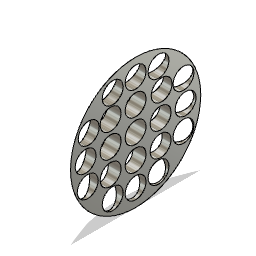
OsmoPod - ZipTie (Autodesk Fusion 360 archive; units mm, degrees)
design "Screen_Cover_12mm"
Autodesk Fusion 360 part; units mm, degrees
sketch "Sketch1" plane through (0, 0, 0) normal (0, 1, 0) x (1, 0, 0)
  line L0 (0, 0) -> (0, 15.875)
  line L1 (0, 0) -> (0, 7.9375)
  line L2 (6.0148, 7.9375) -> (-8.89, 7.9375)
  line L3 (0, 7.9375) -> (-0.254, 7.9375)
  line L4 (0, 7.9375) -> (-1.905, 7.9375)
  line L5 (-1.905, 7.9903) -> (-1.905, 3.048)
  arc A0 (0, 15.875) -> (0, 0) centre (15.584, 7.9375) ccw
  dimension "d1" = 15.875
  dimension "d2" = 1.905
  constraint coincident L0.start L1.start
  constraint vertical L0
  constraint midpoint L0 L1.end
  constraint perpendicular L0 L2
  constraint coincident L2 L3.end
  constraint perpendicular L0 L3
  constraint coincident L2 L4.end
  constraint perpendicular L4 L5
  constraint coincident L4.end A0
  constraint tangent L5 A0
  measures "d1" distance of L0.start L0.end
  measures "d2" distance of L1.end L4.end
revolve "Revolve1" add sketch "Sketch1" angle 360 about axis through (6.0148, 0, -7.9375) along (-1, 0, 0) contours L0 L2 L3 L4 L5 A0
ref_plane "WorkPlane1" through (-2.54, 0, -7.9375) normal (1, 0, 0) x (0, 0, -1)
sketch "Sketch3" plane through (0, 0, 0) normal (1, 0, 0) x (0, 0, -1)
  circle A0 centre (7.9375, 0) radius 7.9375
  circle A1 centre (7.9375, 0) radius 1.2749
  circle A2 centre (7.9375, 2.921) radius 1.2749
  circle A3 centre (7.9375, 5.842) radius 1.2749
  circle A4 centre (7.9375, -2.921) radius 1.2749
  circle A5 centre (7.9375, -5.842) radius 1.2749
  circle A6 centre (10.9855, 0) radius 1.2749
  circle A7 centre (4.8895, 0) radius 1.2749
  circle A8 centre (1.8415, 0) radius 1.2749
  circle A9 centre (14.0335, 0) radius 1.2749
  circle A10 centre (4.8895, 2.921) radius 1.2749
  circle A11 centre (11.1125, 2.921) radius 1.2749
  circle A12 centre (4.8895, -2.921) radius 1.2749
  circle A13 centre (10.9855, -2.921) radius 1.2749
  circle A14 centre (2.2225, 2.794) radius 1.2749
  circle A15 centre (5.1435, 5.588) radius 1.2749
  circle A16 centre (10.7315, 5.588) radius 1.2749
  circle A17 centre (13.7795, 2.794) radius 1.2749
  circle A18 centre (5.1435, -5.588) radius 1.2749
  circle A19 centre (2.0955, -2.794) radius 1.2749
  circle A20 centre (13.7795, -2.794) radius 1.2749
  circle A21 centre (10.7315, -5.588) radius 1.2749
  constraint concentric A0 A1
extrude "Extrude2" cut sketch "Sketch3" against normal blind 3.81 contours A1 | A2 | A3 | A4 | A5 | A6 | A7 | A8 | A9 | A10 | A11 | A12 | A13 | A14 | A15 | A16 | A17 | A18 | A19 | A20 | A21

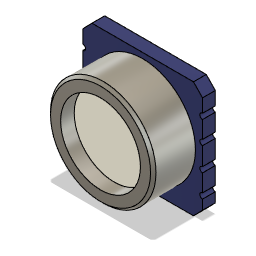
design "MS5803-02BA Package"
Autodesk Fusion 360 part; units mm, degrees
sketch "Sketch1" plane through (0, 0, 0) normal (0, 0, 1) x (1, 0, 0)
  line L0 (2.8, 3.2) -> (-2.8, 3.2)
  line L1 (-2.8, -3.2) -> (2.8, -3.2)
  line L2 (3.0423, 2.9501) -> (-3.0423, -2.9501) construction
  line L3 (-3.0423, 2.9501) -> (3.0423, -2.9501) construction
  circle A0 centre (0, 0) radius 2.2
  line L4 (-2.8, 3.2) -> (-3.3, 2.6844)
  line L5 (3.3, 0) -> (-3.3, 0) construction
  line L6 (0, 3.2) -> (0, -3.2) construction
  line L7 (2.8, 3.2) -> (3.3, 2.6844)
  line L8 (-2.8, -3.2) -> (-3.3, -2.6844)
  line L9 (2.8, -3.2) -> (3.3, -2.6844)
  circle A1 centre (0, 0) radius 2.9075
  line L10 (-2.8, -3.2) -> (-3.3, -3.2) construction
  line L11 (-3.3, -3.2) -> (-3.3, -2) construction
  line L12 (-3.3, -2) -> (-3.3, -0.75) construction
  line L13 (-3.3, -0.75) -> (-3.3, 0.55) construction
  line L14 (-3.3, 0.55) -> (-3.3, 1.8) construction
  arc A2 (-3.3, 0.4) -> (-3.3, 0.7) centre (-3.3, 0.55) ccw
  arc A3 (-3.3, 1.65) -> (-3.3, 1.95) centre (-3.3, 1.8) ccw
  line L15 (-3.3, 2.6844) -> (-3.3, 1.95)
  line L16 (-3.3, 1.65) -> (-3.3, 0.7)
  arc A4 (-3.3, -0.9) -> (-3.3, -0.6) centre (-3.3, -0.75) ccw
  line L17 (-3.3, 0.4) -> (-3.3, -0.6)
  arc A5 (-3.3, -2.15) -> (-3.3, -1.85) centre (-3.3, -2) ccw
  line L18 (-3.3, -0.9) -> (-3.3, -1.85)
  line L19 (-3.3, -2.15) -> (-3.3, -2.6844)
  line L20 (3.3, 2.6844) -> (3.3, 1.95)
  arc A6 (3.3, 1.95) -> (3.3, 1.65) centre (3.3, 1.8) ccw
  arc A7 (3.3, 0.7) -> (3.3, 0.4) centre (3.3, 0.55) ccw
  line L21 (3.3, 1.65) -> (3.3, 0.7)
  line L22 (3.3, 0.4) -> (3.3, -0.6)
  arc A8 (3.3, -0.6) -> (3.3, -0.9) centre (3.3, -0.75) ccw
  arc A9 (3.3, -1.85) -> (3.3, -2.15) centre (3.3, -2) ccw
  line L23 (3.3, -0.9) -> (3.3, -1.85)
  line L24 (3.3, -2.15) -> (3.3, -2.6844)
  dimension "d3" = 4.4
  dimension "d5" = 5.815
  dimension "d13" = 1.2
  dimension "d14" = 1.25
  dimension "d15" = 1.3
  dimension "d16" = 1.25
  dimension "d17" = 0.3
  dimension "d18" = 0.3
  dimension "d19" = 0.3
  dimension "d20" = 0.3
  constraint perpendicular L0 L15
  constraint parallel L0 L1
  constraint horizontal L0
  constraint coincident L2 A0.centre
  constraint coincident L3 A0.centre
  constraint coincident A0.centre A1.centre
  constraint perpendicular L3 L4
  constraint symmetric L0.end L6 L0.start
  constraint symmetric L4.end L6 L7.end
  constraint symmetric L0.end L5 L1.start
  constraint symmetric L4.end L5 L8.end
  constraint symmetric L5 L0.start L1.end
  constraint symmetric L5 L7.end L9.end
  constraint coincident L0 L6.start
  constraint coincident L7 L2.start
  constraint coincident L9 L3.end
  constraint coincident L1 L6.end
  constraint coincident L8 L2.end
  constraint coincident L5.end L15
  constraint coincident L4 L3.start
  constraint perpendicular L10 L15
  constraint perpendicular L10 L11
  constraint parallel L12 L15
  constraint parallel L13 L15
  constraint parallel L14 L15
  constraint coincident L14.end A3.centre
  constraint coincident L13.end L14.start
  constraint coincident L12.end L13.start
  constraint coincident L11.end L12.start
  constraint coincident A2.start L15
  constraint collinear L15 L17
  constraint coincident L14 A3.start
  constraint collinear L15 L16
  constraint coincident L13 A4.end
  constraint coincident L12 A4.start
  constraint collinear L17 L18
  constraint coincident L12 A5.end
  constraint coincident L11 A5.start
  constraint collinear L18 L19
  constraint symmetric L6 L8.end L9.end
  constraint symmetric L6 A2.end A7.start
  constraint symmetric L6 A2.start A7.end
  constraint symmetric L6 A2 A7
  constraint symmetric L6 A3.end L20.end
  constraint symmetric L6 A3.start A6.end
  constraint symmetric L6 A3 A6
  constraint symmetric L6 A4.end L22.end
  constraint symmetric L6 A4.start A8.end
  constraint symmetric L6 A4 A8
  constraint symmetric L6 A5.end A9.start
  constraint symmetric L6 A5.start A9.end
  constraint symmetric L6 A5 A9
  measures "d3" diameter of A0
  measures "d5" diameter of A1
  measures "d13" distance of L10.end L11.end
  measures "d14" distance of L11.end L12.end
  measures "d15" distance of L12.end L13.end
  measures "d16" distance of L13.end L14.end
  measures "d17" diameter of A3
  measures "d18" diameter of A2
  measures "d19" diameter of A4
  measures "d20" diameter of A5
extrude "Extrude1" add sketch "Sketch1" along normal blind 0.705 contours L0 L1 L4 L7 L8 L9 A2 A3 L15 L16 A4 L17 A5 L18 L19 L20 A6 A7 L21 L22 A8 A9 L23 L24 | A0 | A1
extrude "Extrude2" add sketch "Sketch1" along normal blind 3.03 contours A1
chamfer "Chamfer1" distance 0.15 angle 45 1 edges at (-2.7107, -1.0514, 3.03)
extrude "Extrude3" add 1 faces at (0.294, -0.2907, 0.705) along direction (0, 0, 1) blind 1.575
equation "d6 = 0.635 mm + 0.07 mm"
equation "d8 = 2.88 mm + 0.15 mm"
equation "d11 = 2.325 mm - 0.75 mm"
equation "d17 = ( 0.15 * 2 ) * 1 mm"

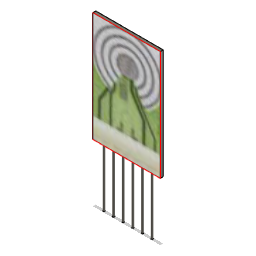
design "LFS1107"
Autodesk Fusion 360 part; units mm, degrees
sketch "Sketch1" plane through (0, 0, 0) normal (0, 0, 1) x (1, 0, 0)
  line L0 (0, 0) -> (7, 0)
  line L1 (7, 0) -> (7, 11.4)
  line L2 (7, 11.4) -> (0, 11.4)
  line L3 (0, 11.4) -> (0, 0)
  dimension "d1" = 7
  dimension "d2" = 11.4
  constraint horizontal L0
  constraint vertical L1
  constraint horizontal L2
  constraint vertical L3
  constraint coincident L0.start L3.end
  measures "d1" distance of L0.start L0.end
  measures "d2" distance of L0.start L2.end
extrude "Extrude1" add sketch "Sketch1" along normal blind 0.3
cylinder "CylinderPrimitive1" add diameter 0.2 height 0.05 placed x (1, 0, 0) y (0, 0, 1) z (0, -1, 0) at (0.5, 0, 0.15)
delete_face "DeleteFace1" 1 faces at (0.5995, -0.0333, 0.14)
sketch "Sketch3" plane through (0, 0, 0) normal (0, -1, 0) x (1, 0, 0)
  line L0 (0, 0) -> (7, 0)
  line L1 (7, 0) -> (7, 0.3)
  line L2 (7, 0.3) -> (0, 0.3)
  line L3 (0, 0.3) -> (0, 0)
  circle A0 centre (1, 0.15) radius 0.1
  circle A1 centre (2, 0.15) radius 0.1
  circle A2 centre (3, 0.15) radius 0.1
  circle A3 centre (4, 0.15) radius 0.1
  circle A4 centre (5, 0.15) radius 0.1
  circle A5 centre (6, 0.15) radius 0.1
  dimension "d7" = 1
  dimension "d10" = 5
  dimension "d11" = 0
  measures "d7" distance of L3 A0.centre
extrude "Extrude2" add sketch "Sketch3" along normal blind 6 contours A0 | A1 | A2 | A3 | A4 | A5
